Autodesk Fusion 360 part; units mm, degrees
(part 5 of 7)
sketch "Sketch93" plane through (0, 0, 13.6) normal (0, 0, -1) x (1, 0, 0)
  circle A0 centre (117.65, -41.45) radius 3.85
  circle A1 centre (102.6547, -56.4453) radius 2.35
  circle A2 centre (110.15, -33.95) radius 3.85
  circle A3 centre (117.6453, -56.4453) radius 2.35
  circle A4 centre (110.15, -48.95) radius 3.85
  circle A5 centre (102.65, -41.45) radius 3.85
  circle A6 centre (110.2363, -20.8316) radius 2.5
  circle A7 centre (110.15, -62.1) radius 2.5
  line L0 (119.9, -7.9) -> (124.4, -7.9)
  line L1 (124.4, -7.9) -> (124.4, -12.9)
  line L2 (124.4, -12.9) -> (119.9, -12.9)
  line L3 (119.9, -12.9) -> (119.9, -7.9)
  line L4 (118.9, -24.9) -> (119.9, -24.9)
  line L5 (119.9, -24.9) -> (119.9, -19.9)
  line L6 (119.9, -19.9) -> (124.4, -19.9)
  line L7 (124.4, -19.9) -> (124.4, -24.9)
  line L8 (124.4, -24.9) -> (124.4, -25.9)
  line L9 (124.4, -25.9) -> (118.9, -25.9)
  line L10 (118.9, -25.9) -> (118.9, -24.9)
  line L11 (95.9, -0.9) -> (95.9, -24.9)
  line L12 (95.9, -24.9) -> (101.9, -24.9)
  line L13 (101.9, -24.9) -> (101.9, -25.9)
  line L14 (101.9, -25.9) -> (95.9, -25.9)
  line L15 (95.9, -25.9) -> (95.9, -77.2)
  line L16 (95.9, -77.2) -> (75.9, -77.2)
  line L17 (75.9, -77.2) -> (75.9, -85.1)
  line L18 (75.9, -85.1) -> (106.4, -85.1)
  arc A8 (106.4, -85.1) -> (126.4, -65.1) centre (106.4, -65.1) ccw
  line L19 (126.4, -65.1) -> (126.4, 4.1)
  line L20 (126.4, 4.1) -> (124.4, 4.1)
  line L21 (124.4, 4.1) -> (124.4, -0.9)
  line L22 (124.4, -0.9) -> (119.9, -0.9)
  line L23 (119.9, -0.9) -> (119.9, 4.1)
  line L24 (119.9, 4.1) -> (118.9, 4.1)
  line L25 (118.9, 4.1) -> (118.9, 1.6)
  line L26 (118.9, 1.6) -> (118.9, -0.9)
  line L27 (118.9, -0.9) -> (116.4, -0.9)
  line L28 (116.4, -0.9) -> (113.9, -0.9)
  line L29 (113.9, -0.9) -> (113.9, 1.2)
  line L30 (113.9, 1.2) -> (112.9, 1.2)
  line L31 (112.9, 1.2) -> (112.9, -0.9)
  line L32 (112.9, -0.9) -> (107.9, -0.9)
  line L33 (107.9, -0.9) -> (107.9, 1.2)
  line L34 (107.9, 1.2) -> (100.8678, 1.2)
  line L35 (100.8678, 1.2) -> (100.8704, -0.9)
  line L36 (100.8704, -0.9) -> (98.4, -0.9)
  line L37 (98.4, -0.9) -> (95.9, -0.9)
  line L38 (126.4, -65.1) -> (126.4, 4.1)
  arc A9 (106.4, -85.1) -> (126.4, -65.1) centre (106.4, -65.1) ccw
  line L39 (75.9, -85.1) -> (106.4, -85.1)
  line L40 (-2, -85.1) -> (75.9, -85.1)
  line L41 (-2, -85.1) -> (-12.5, -85.1)
  arc A10 (-32.5, -65.1) -> (-12.5, -85.1) centre (-12.5, -65.1) ccw
  arc A11 (-31.5, -65.1) -> (-12.5, -84.1) centre (-12.5, -65.1) ccw
  line L42 (-12.5, -84.1) -> (-6.5, -84.1)
  line L43 (-31.5, -59.1) -> (-31.5, -65.1)
  line L44 (-32.5, -65.1) -> (-32.5, -25.2)
  line L45 (-32.5, 4.1) -> (-32.5, -25.2)
  line L46 (-31.5, 4.1) -> (-31.5, -25.9)
  line L47 (-32.5, 25.3) -> (-32.5, 4.1)
  arc A12 (-22.5, 35.3) -> (-32.5, 25.3) centre (-22.5, 25.3) ccw
  line L48 (116.4, 35.3) -> (-22.5, 35.3)
  arc A13 (126.4, 25.3) -> (116.4, 35.3) centre (116.4, 25.3) ccw
  line L49 (126.4, 4.1) -> (126.4, 25.3)
  line L50 (46.95, 35.3) -> (46.95, 14.5814) construction
  arc A14 (106.4, -84.1) -> (125.4, -65.1) centre (106.4, -65.1) ccw
  line L51 (-31.5, -59.1) -> (-31.5, -25.9)
  line L52 (-32.5, 25.3) -> (-31.5, 25.3) construction
  line L53 (-31.5, 25.3) -> (-31.5, 4.1)
  line L54 (116.4, 35.3) -> (116.4, 34.3) construction
  line L55 (116.4, 34.3) -> (-22.5, 34.3)
  arc A15 (-22.5, 34.3) -> (-31.5, 25.3) centre (-22.5, 25.3) ccw
  arc A16 (125.4, 25.3) -> (116.4, 34.3) centre (116.4, 25.3) ccw
  line L56 (125.4, 4.1) -> (125.4, -25.9)
  line L57 (125.4, 25.3) -> (125.4, 4.1)
  line L58 (125.4, -59.1) -> (125.4, -25.9)
  line L59 (125.4, -65.1) -> (125.4, -59.1)
  line L60 (106.4, -84.1) -> (-6.5, -84.1)
  line L61 (126.4, -65.1) -> (125.4, -65.1)
  line L62 (106.4, -85.1) -> (106.4, -84.1)
  line L63 (-12.5, -85.1) -> (-12.5, -84.1)
  line L64 (-32.5, -65.1) -> (-31.5, -65.1)
  line L65 (116.4, 35.3) -> (116.4, 34.3)
  line L66 (-22.5, 35.3) -> (-22.5, 34.3)
  dimension "d636" = 1
  dimension "d637" = 1
  constraint midpoint L48 L50.start
  constraint perpendicular L48 L50
  constraint symmetric A11.start L50 A14.end
  constraint symmetric A11.end L50 A14.start
  constraint symmetric A11 L50 A14
  constraint coincident L43.start L51.start
  constraint coincident L46.end L51.end
  constraint coincident L47.start A12.end
  constraint perpendicular L47 L52
  constraint concentric A12 A15
  constraint coincident L46.start L53.end
  constraint coincident L48.start A13.end
  constraint perpendicular L48 L54
  constraint tangent L55 A15
  constraint symmetric L46.start L50 L56.start
  constraint symmetric L46.end L50 L56.end
  constraint symmetric L50 L43.start L58.start
  constraint symmetric L50 L46.end L56.end
  constraint symmetric L50 L52.end A16.start
  constraint symmetric L50 L46.start L56.start
  constraint symmetric L50 L55.end L54.end
  constraint symmetric L50 A15 A16
  constraint coincident L42.end L60.end
  constraint coincident A8.end L19.start
  constraint coincident L18.end A8.start
  constraint coincident L41.end A10.end
  constraint coincident A11.end L42.start
  constraint coincident A10.start L44.start
  constraint coincident A11.start L43.end
  constraint coincident A12.start L48.end
  measures "d636" distance of L47.start L52.end
  measures "d637" distance of L48.start L54.end
extrude "Extrude79" add sketch "Sketch93" along normal blind 22 contours L19 L20 L38 L56 L58 L59 L61 | L43 L44 L45 L46 L47 A12 L51 L53 A15 L64 L66 | L20 A13 L49 A16 L57 L65 bodies 3
extrude "Extrude80" add 1 faces at (33.342, 24.9132, -5.7) along direction (0, 0, -1) blind 8 on bodies 2 bodies 2
extrude "Extrude82" add 7 faces at (126.0667, 11.9, -8.4) (114.6093, -1.7242, -8.4) (118.1907, -25.4242, -8.4) (18.7093, 81.2742, -8.4) (-20.7093, -1.7242, -8.4) (-20.7093, -25.1758, -8.4) (-31.8333, 28.7333, -8.4) along direction (0, 0, -1) blind 8 on bodies 3 bodies 3
sketch "Sketch95" plane through (-32.5, 0, 0) normal (-1, 0, 0) x (0, -1, 0)
  line L0 (25.3, -16.4) -> (25.3, 14.6)
  line L1 (25.3, 14.6) -> (4.1, 14.6)
  line L2 (4.1, 14.6) -> (4.1, 13.6)
  line L3 (4.1, 13.6) -> (-25.2, 13.6)
  line L4 (-25.2, 13.6) -> (-25.2, -16.4)
  line L5 (-25.2, -16.4) -> (25.3, -16.4)
  line L6 (-11.4882, 13.6) -> (30.9382, 13.6) construction
  line L7 (-11.4882, 13.6) -> (-13.9882, 13.6)
  line L8 (-11.4882, 13.6) -> (-8.9882, 13.6)
  line L9 (18.5118, -16.4) -> (21.0118, -16.4)
  line L10 (18.5118, -16.4) -> (16.0118, -16.4)
  line L11 (-13.9882, 13.6) -> (16.0118, -16.4)
  line L12 (-8.9882, 13.6) -> (21.0118, -16.4)
  dimension "d658" = 2.5
  dimension "d659" = 2.5
  dimension "d660" = 2.5
  dimension "d661" = 2.5
  constraint horizontal L6
  constraint coincident L3 L6.start
  constraint coincident L5 L9.start
  constraint parallel L3 L7
  constraint parallel L6 L8
  constraint parallel L5 L9
  constraint parallel L5 L10
  measures "d658" distance of L6.start L7.end
  measures "d659" distance of L6.start L8.end
  measures "d660" distance of L9.start L9.end
  measures "d661" distance of L9.start L10.end
extrude "Extrude84" add sketch "Sketch95" along normal blind 1 contours L3 L5 L7 L8 L9 L10 L11 L12 bodies 3 6 8
fillet "Fillet7" radius 5 1 edges at (-32.5, -6.0118, -1.4) on bodies 3
fillet "Fillet8" radius 8.5 1 edges at (-33.5, -6.0118, -1.4) on bodies 3
fillet "Fillet9" radius 5 1 edges at (-32.5, -1.0118, -1.4) on bodies 3
fillet "Fillet10" radius 8.5 1 edges at (-33.5, -1.0118, -1.4) on bodies 3
sketch "Sketch97" plane through (0, 0, 15.6) normal (0, 0, 1) x (-1, 0, 0)
  arc A0 (31.5, 25.3) -> (27.4749, 32.8) centre (22.5, 25.3) ccw
  line L0 (27.4749, 32.8) -> (15.9888, 32.8)
  line L1 (15.9888, 32.8) -> (17.8764, 30.7591)
  arc A1 (15.9888, 31.4975) -> (17.8764, 30.7591) centre (16.1, 29) ccw
  line L2 (15.9888, 31.4975) -> (15.9888, 32.8)
  line L3 (15.9888, 32.8) -> (-121.3749, 32.8)
  arc A2 (-121.3749, 32.8) -> (-125.4, 25.3) centre (-116.4, 25.3) ccw
  line L4 (-125.4, 25.3) -> (-125.4, -65.1)
  arc A3 (-125.4, -65.1) -> (-106.4, -84.1) centre (-106.4, -65.1) ccw
  line L5 (-106.4, -84.1) -> (12.5, -84.1)
  arc A4 (12.5, -84.1) -> (31.5, -65.1) centre (12.5, -65.1) ccw
  line L6 (31.5, -65.1) -> (31.5, -25.2)
  line L7 (31.5, -25.2) -> (31.5, 25.3)
  line L8 (0, 4.1) -> (0, -75.1)
  line L9 (0, -75.1) -> (-93.9, -75.1)
  line L10 (-93.9, -75.1) -> (-93.9, 4.1)
  line L11 (-93.9, 4.1) -> (0, 4.1)
  circle A5 centre (-102.6547, -56.4453) radius 2.35
  circle A6 centre (-117.6453, -56.4453) radius 2.35
  circle A7 centre (-110.15, -33.95) radius 3.85
  circle A8 centre (-102.65, -41.45) radius 3.85
  circle A9 centre (-117.65, -41.45) radius 3.85
  circle A10 centre (-110.15, -48.95) radius 3.85
  arc A11 (-46.45, -79.6) -> (-47.45, -79.6) centre (-46.95, -79.6) ccw
  line L12 (-46.45, -79.6) -> (-45.65, -79.6)
  arc A12 (-45.65, -80.6) -> (-45.65, -79.6) centre (-45.65, -80.1) ccw
  line L13 (-45.65, -80.6) -> (-46.45, -80.6)
  arc A13 (-47.45, -80.6) -> (-46.45, -80.6) centre (-46.95, -80.6) ccw
  line L14 (-47.45, -80.6) -> (-48.25, -80.6)
  arc A14 (-48.25, -79.6) -> (-48.25, -80.6) centre (-48.25, -80.1) ccw
  line L15 (-48.25, -79.6) -> (-47.45, -79.6)
  line L16 (-98.8996, 12.7) -> (-88.8996, 12.7)
  arc A15 (-88.9, 10.7) -> (-88.8996, 12.7) centre (-88.9, 11.7) ccw
  line L17 (-88.9, 10.7) -> (-98.9, 10.7)
  arc A16 (-98.8996, 12.7) -> (-98.9, 10.7) centre (-98.9, 11.7) ccw
  line L18 (-85.7348, 14.7) -> (-102.0652, 14.7)
  arc A17 (-102.0652, 16.7) -> (-102.0652, 14.7) centre (-102.0652, 15.7) ccw
  line L19 (-102.0652, 16.7) -> (-85.7348, 16.7)
  arc A18 (-85.7348, 14.7) -> (-85.7348, 16.7) centre (-85.7348, 15.7) ccw
  arc A19 (-102.0652, 24.7) -> (-102.0652, 22.7) centre (-102.0652, 23.7) ccw
  line L20 (-102.0652, 24.7) -> (-85.7348, 24.7)
  arc A20 (-85.7348, 22.7) -> (-85.7348, 24.7) centre (-85.7348, 23.7) ccw
  line L21 (-85.7348, 22.7) -> (-102.0652, 22.7)
  arc A21 (-98.9, 28.7) -> (-98.9004, 26.7) centre (-98.9, 27.7) ccw
  line L22 (-98.9, 28.7) -> (-88.9, 28.7)
  arc A22 (-88.8996, 26.7) -> (-88.9, 28.7) centre (-88.9, 27.7) ccw
  line L23 (-88.8996, 26.7) -> (-98.9004, 26.7)
  arc A23 (-102.9, 20.7) -> (-102.9, 18.7) centre (-102.9, 19.7) ccw
  line L24 (-102.9, 20.7) -> (-84.9, 20.7)
  arc A24 (-84.9, 18.7) -> (-84.9, 20.7) centre (-84.9, 19.7) ccw
  line L25 (-84.9, 18.7) -> (-102.9, 18.7)
  line L26 (8.1652, 14.7) -> (-8.1652, 14.7)
  arc A25 (-8.1652, 16.7) -> (-8.1652, 14.7) centre (-8.1652, 15.7) ccw
  line L27 (-8.1652, 16.7) -> (8.1652, 16.7)
  arc A26 (8.1652, 14.7) -> (8.1652, 16.7) centre (8.1652, 15.7) ccw
  arc A27 (9, 18.7) -> (9, 20.7) centre (9, 19.7) ccw
  line L28 (9, 18.7) -> (-9, 18.7)
  arc A28 (-9, 20.7) -> (-9, 18.7) centre (-9, 19.7) ccw
  line L29 (-9, 20.7) -> (9, 20.7)
  line L30 (-8.1652, 24.7) -> (8.1652, 24.7)
  arc A29 (8.1652, 22.7) -> (8.1652, 24.7) centre (8.1652, 23.7) ccw
  line L31 (8.1652, 22.7) -> (-8.1652, 22.7)
  arc A30 (-8.1652, 24.7) -> (-8.1652, 22.7) centre (-8.1652, 23.7) ccw
  arc A31 (5.0004, 26.7) -> (5, 28.7) centre (5, 27.7) ccw
  line L32 (5.0004, 26.7) -> (-4.9996, 26.7)
  arc A32 (-5, 28.7) -> (-4.9996, 26.7) centre (-5, 27.7) ccw
  line L33 (-5, 28.7) -> (5, 28.7)
  arc A33 (5, 10.7) -> (5.0004, 12.7) centre (5, 11.7) ccw
  line L34 (5, 10.7) -> (-5, 10.7)
  arc A34 (-5.0004, 12.7) -> (-5, 10.7) centre (-5, 11.7) ccw
  line L35 (-5.0004, 12.7) -> (5.0004, 12.7)
  line L36 (-34.2, 32.4) -> (-34.2, 30.4)
  line L37 (-34.2, 30.4) -> (-27.2, 30.4)
  line L38 (-27.2, 30.4) -> (-27.2, 10)
  arc A35 (-29.2, 8) -> (-27.2, 10) centre (-29.2, 10) ccw
  line L39 (-29.2, 8) -> (-64.7, 8)
  arc A36 (-66.7, 10) -> (-64.7, 8) centre (-64.7, 10) ccw
  line L40 (-66.7, 10) -> (-66.7, 30.4)
  line L41 (-66.7, 30.4) -> (-59.7, 30.4)
  line L42 (-59.7, 30.4) -> (-59.7, 32.4)
  line L43 (-59.7, 32.4) -> (-34.2, 32.4)
  line L44 (13, -32.2) -> (19.5, -32.2)
  line L45 (19.5, -32.2) -> (19.5, -38.2)
  line L46 (19.5, -38.2) -> (25.5, -38.2)
  line L47 (25.5, -38.2) -> (25.5, -44.7)
  line L48 (25.5, -44.7) -> (19.5, -44.7)
  line L49 (19.5, -44.7) -> (19.5, -50.7)
  line L50 (19.5, -50.7) -> (13, -50.7)
  line L51 (13, -50.7) -> (13, -44.7)
  line L52 (13, -44.7) -> (7, -44.7)
  line L53 (7, -44.7) -> (7, -38.2)
  line L54 (7, -38.2) -> (13, -38.2)
  line L55 (13, -38.2) -> (13, -32.2)
  circle A37 centre (10.8119, -62.3239) radius 1.5
  circle A38 centre (16.25, -62.1) radius 0.4
  line L56 (16.25, -62.1) -> (16.25, -66.288) construction
  line L57 (10.8119, -62.3239) -> (16.25, -62.3239) construction
  line L58 (16.25, -62.3239) -> (21.688, -62.3239) construction
  line L59 (21.688, -62.3239) -> (21.688, -60.8239) construction
  line L60 (20.188, -62.3239) -> (20.188, -59.3239)
  line L61 (23.188, -62.3239) -> (23.188, -59.3239)
  arc A39 (20.188, -62.3239) -> (23.188, -62.3239) centre (21.688, -62.3239) ccw
  arc A40 (23.188, -59.3239) -> (20.188, -59.3239) centre (21.688, -59.3239) ccw
  dimension "d674" = 5.438
  dimension "d675" = 3
  dimension "d676" = 3
  constraint coincident A38.centre L56.start
  constraint vertical L56
  constraint coincident A37.centre L57.start
  constraint coincident L56 L57.end
  constraint perpendicular L56 L57
  constraint perpendicular L56 L58
  constraint coincident L58.end L59.start
  constraint perpendicular L58 L59
  constraint tangent A39 A40
  constraint coincident L58 L60.start
  constraint tangent L60 A40
  constraint tangent L61 A40
  constraint parallel L60 L61
  measures "d674" distance of L57.end L58.end
  measures "d675" diameter of A39
  measures "d676" distance of L58.end A40.centre
extrude "Extrude85" cut sketch "Sketch97" against normal blind 1 contours L60 L61 A39 A40 bodies 3
sketch "Sketch98" plane through (126.4, 0, 0) normal (1, 0, 0) x (0, 1, 0)
  line L0 (65.1, 13.6) -> (65.1, 14.6)
  line L1 (65.1, 14.6) -> (-25.3, 14.6)
  line L2 (-25.3, 14.6) -> (-25.3, -16.4)
  line L3 (-25.3, -16.4) -> (65.1, -16.4)
  line L4 (65.1, -16.4) -> (65.1, 13.6)
  line L5 (-21.0118, -16.4) -> (-16.0118, -16.4)
  line L6 (13.9, 13.6) -> (8.9882, 13.6)
  line L7 (8.9882, 13.6) -> (-21.0118, -16.4)
  line L8 (13.9, 13.6) -> (-16.0118, -16.4)
  point P0 (-21.0118, -16.4)
  point P1 (-16.0118, -16.4)
  point P2 (13.9, 13.6)
  point P3 (8.9882, 13.6)
  constraint coincident P0 L5.start
  constraint coincident P1 L5.end
  constraint coincident P2 L6.start
  constraint coincident P3 L6.end
extrude "Extrude86" add sketch "Sketch98" along normal blind 1 contours L3 L5 L6 L7 L8 bodies 3 6 8
fillet "Fillet13" radius 5 1 edges at (126.4, -6.0118, -1.4) on bodies 3
fillet "Fillet14" radius 8.5 1 edges at (127.4, -6.0118, -1.4) on bodies 3
fillet "Fillet15" radius 5 1 edges at (126.4, -1.0559, -1.4) on bodies 3
fillet "Fillet16" radius 8.5 1 edges at (127.4, -1.0559, -1.4) on bodies 3
sketch "Sketch102" plane through (0, 0, 10) normal (0, 0, -1) x (1, 0, 0)
  line L0 (-31.5, 25.3) -> (-31.5, 4.1)
  line L1 (-31.5, 4.1) -> (-25, 4.1)
  line L2 (-25, 4.1) -> (-25, 1.6)
  arc A0 (-23, 4.0495) -> (-25, 1.6) centre (-22.5, 1.6) ccw
  line L3 (-23, 4.0495) -> (-23, 22.8505)
  arc A1 (-22, 22.8505) -> (-23, 22.8505) centre (-22.5, 25.3) ccw
  line L4 (-22, 22.8505) -> (-22, 4.0495)
  arc A2 (-20, 1.6) -> (-22, 4.0495) centre (-22.5, 1.6) ccw
  line L5 (-20, 1.6) -> (-20, 2)
  line L6 (-20, 2) -> (-7, 2)
  line L7 (-7, 2) -> (-7, 4.1)
  line L8 (-7, 4.1) -> (-4.5, 4.1)
  line L9 (-4.5, 4.1) -> (-2, 4.1)
  line L10 (-2, 4.1) -> (0, 4.1)
  line L11 (0, 4.1) -> (0, 5.7)
  arc A3 (13.4164, 23.7) -> (0, 5.7) centre (0, 19.7) ccw
  line L12 (13.4164, 23.7) -> (27.2, 23.7)
  line L13 (27.2, 23.7) -> (27.2, 33.9)
  line L14 (27.2, 33.9) -> (66.7, 33.9)
  line L15 (66.7, 33.9) -> (66.7, 23.7)
  line L16 (66.7, 23.7) -> (80.4836, 23.7)
  arc A4 (93.9, 5.7) -> (80.4836, 23.7) centre (93.9, 19.7) ccw
  line L17 (93.9, 5.7) -> (93.9, 4.1)
  line L18 (93.9, 4.1) -> (95.9, 4.1)
  line L19 (95.9, 4.1) -> (98.4, 4.1)
  line L20 (98.4, 4.1) -> (100.9, 4.1)
  line L21 (100.9, 4.1) -> (100.9, 2)
  line L22 (100.9, 2) -> (113.9322, 2)
  arc A5 (115.9, 4.0495) -> (113.9322, 2) centre (116.4, 1.6) ccw
  line L23 (115.9, 4.0495) -> (115.9, 22.8505)
  arc A6 (116.9, 22.8505) -> (115.9, 22.8505) centre (116.4, 25.3) ccw
  line L24 (116.9, 22.8505) -> (116.9, 4.0495)
  arc A7 (118.9, 1.6) -> (116.9, 4.0495) centre (116.4, 1.6) ccw
  line L25 (118.9, 1.6) -> (118.9, 4.1)
  line L26 (118.9, 4.1) -> (125.4, 4.1)
  line L27 (125.4, 4.1) -> (125.4, 25.3)
  arc A8 (125.4, 25.3) -> (116.4, 34.3) centre (116.4, 25.3) ccw
  line L28 (116.4, 34.3) -> (116.4, 35.3)
  line L29 (116.4, 35.3) -> (-22.5, 35.3)
  line L30 (-22.5, 35.3) -> (-22.5, 34.3)
  arc A9 (-22.5, 34.3) -> (-31.5, 25.3) centre (-22.5, 25.3) ccw
  line L31 (116.4, 35.3) -> (96.4, 35.3)
  line L32 (96.4, 35.3) -> (96.4, 34.3)
  line L33 (96.4, 34.3) -> (116.4, 34.3)
  line L34 (116.4, 34.3) -> (116.4, 35.3)
  line L35 (46.95, 35.3) -> (46.95, 48.5522) construction
  line L36 (46.95, 35.3) -> (46.95, 48.5522) construction
  line L37 (-22.5, 35.3) -> (-2.5, 35.3)
  line L38 (-2.5, 35.3) -> (-2.5, 34.3)
  line L39 (-2.5, 34.3) -> (-22.5, 34.3)
  line L40 (-22.5, 34.3) -> (-22.5, 35.3)
  dimension "d693" = 20
  dimension "d694" = 1
  constraint coincident L28.end L29.start
  constraint perpendicular L28 L31
  constraint perpendicular L31 L32
  constraint coincident A8.end L28.start
  constraint midpoint L29 L35.start
  constraint perpendicular L29 L35
  constraint symmetric L28.end L35 L29.end
  constraint symmetric L31.end L35 L37.end
  constraint symmetric L32.end L35 L38.end
  constraint symmetric A8.end L35 L30.end
  constraint symmetric L36.start L35 L35.start
  constraint symmetric L36.end L35 L35.end
  measures "d693" distance of L28.end L31.end
  measures "d694" distance of L31.end L32.end
extrude "Extrude87" add sketch "Sketch102" along normal blind 26.4 contours L29 L30 L37 L38 L39 L40 | L28 L29 L31 L32 L33 L34 bodies 3 6 8
sketch "ExportDXF" plane through (0, 0, -16.4) normal (0, 0, -1) x (1, 0, 0)
  circle A0 centre (116.4, 1.6) radius 0.4
  circle A1 centre (116.4, 1.6) radius 2.5
  spline S0 degree 3 poles (121.3749, 32.8) (121.4016, 32.8) (121.4257, 32.8021) (121.4681, 32.811) (121.489, 32.8182) (121.521, 32.8394) (121.5326, 32.8506) (121.5513, 32.8783) (121.5579, 32.8938) (121.5687, 32.9351) (121.5705, 32.9623) (121.568, 33.0372) (121.5571, 33.0944) (121.5047, 33.2719) (121.442, 33.4168) (121.2247, 33.772) (121.0595, 33.976) (120.605, 34.3502) (120.3486, 34.4924) (120.0657, 34.6039) knots 1.719139 1.719139 1.719139 1.719139 1.741292 1.741292 1.762806 1.762806 1.778603 1.778603 1.794207 1.794207 1.817491 1.817491 1.860621 1.860621 1.939646 1.939646 2.038469 2.038469 2.13754 2.13754 2.13754 2.13754
  arc A2 (126.4, 25.3) -> (120.0657, 34.6039) centre (116.4, 25.3) ccw
  line L0 (126.4, 25.3) -> (125.4, 25.3)
  arc A3 (125.4, 25.3) -> (121.3749, 32.8) centre (116.4, 25.3) ccw
  circle A4 centre (98.4, 1.6) radius 0.4
  circle A5 centre (110.2363, -20.8316) radius 2.5
  circle A6 centre (110.2363, -20.8316) radius 2.5
  line L1 (115.9, 22.8505) -> (115.9, 4.0495)
  line L2 (115.9, 4.0495) -> (115.9, 22.8505)
  circle A7 centre (102.6547, -56.4453) radius 2.35
  circle A8 centre (102.6547, -56.4453) radius 2.35
  line L3 (-25, 1.6) -> (-25, -0.9)
  line L4 (-25, -0.9) -> (-25, 1.6)
  circle A9 centre (117.6453, -56.4453) radius 2.35
  circle A10 centre (117.6453, -56.4453) radius 2.35
  circle A11 centre (98.4, 1.6) radius 0.4
  circle A12 centre (98.4, 1.6) radius 0.4
  circle A13 centre (116.4, 25.3) radius 0.4
  circle A14 centre (116.4, 25.3) radius 2.5
  arc A15 (106.4, -85.1) -> (126.4, -65.1) centre (106.4, -65.1) ccw
  arc A16 (106.4, -85.1) -> (126.4, -65.1) centre (106.4, -65.1) ccw
  line L5 (96.4, 34.3) -> (116.4, 34.3)
  line L6 (116.4, 34.3) -> (96.4, 34.3)
  line L7 (-22.4996, -0.9) -> (-25, -0.9)
  line L8 (-25, -0.9) -> (-22.4996, -0.9)
  line L9 (-25, 4.1) -> (-25, 1.6)
  line L10 (-25, 1.6) -> (-25, 4.1)
  circle A17 centre (116.4, 1.6) radius 2.5
  arc A18 (113.9322, 2) -> (113.9322, 1.2) centre (116.4, 1.6) ccw
  arc A19 (113.9322, 1.2) -> (116.4, -0.9) centre (116.4, 1.6) ccw
  arc A20 (116.4, -0.9) -> (118.9, 1.6) centre (116.4, 1.6) ccw
  arc A21 (118.9, 1.6) -> (116.9, 4.0495) centre (116.4, 1.6) ccw
  arc A22 (116.9, 4.0495) -> (115.9, 4.0495) centre (116.4, 1.6) ccw
  arc A23 (115.9, 4.0495) -> (113.9322, 2) centre (116.4, 1.6) ccw
  line L11 (-26, 4.1) -> (-26, -0.9)
  line L12 (-26, -0.9) -> (-26, 4.1)
  circle A24 centre (116.4, 1.6) radius 0.4
  arc A25 (116.4, 2) -> (116.3992, 1.2) centre (116.4, 1.6) ccw
  arc A26 (116.3992, 1.2) -> (116.4, 2) centre (116.4, 1.6) ccw
  circle A27 centre (110.2363, -20.8316) radius 0.4
  circle A28 centre (110.2363, -20.8316) radius 2.5
  line L13 (116.9, 4.0495) -> (116.9, 22.8505)
  line L14 (116.9, 22.8505) -> (116.9, 4.0495)
  line L15 (125.4, 4.1) -> (118.9, 4.1)
  line L16 (118.9, 4.1) -> (119.9, 4.1)
  line L17 (119.9, 4.1) -> (124.4, 4.1)
  line L18 (124.4, 4.1) -> (125.4, 4.1)
  line L19 (-19, -6.9) -> (-14, -6.9)
  line L20 (-14, -6.9) -> (-14, -1.9)
  line L21 (-14, -1.9) -> (-19, -1.9)
  line L22 (-19, -1.9) -> (-19, -6.9)
  arc A29 (113.9322, 2) -> (113.9322, 1.2) centre (116.4, 1.6) ccw
  line L23 (113.9322, 2) -> (100.9, 2)
  line L24 (100.9, 2) -> (100.9, 1.6)
  arc A30 (100.8678, 1.2) -> (100.9, 1.6) centre (98.4, 1.6) ccw
  line L25 (100.8678, 1.2) -> (113.9322, 1.2)
  arc A31 (125.4, 25.3) -> (116.4, 34.3) centre (116.4, 25.3) ccw
  arc A32 (125.4, 25.3) -> (116.4, 34.3) centre (116.4, 25.3) ccw
  line L26 (-30.5, 4.1) -> (-30.5, -0.9)
  line L27 (-30.5, -0.9) -> (-26, -0.9)
  line L28 (-26, -0.9) -> (-26, 4.1)
  line L29 (-26, 4.1) -> (-30.5, 4.1)
  line L30 (113.9322, 2) -> (100.9, 2)
  line L31 (100.9, 2) -> (113.9322, 2)
  line L32 (-25, 1.6) -> (-25, -0.9)
  line L33 (-25, -0.9) -> (-22.4996, -0.9)
  arc A33 (-25, 1.6) -> (-22.4996, -0.9) centre (-22.5, 1.6) ccw
  line L34 (-26, -6.9) -> (-26, -1.9)
  line L35 (-26, -1.9) -> (-30.5, -1.9)
  line L36 (-30.5, -1.9) -> (-30.5, -6.9)
  line L37 (-30.5, -6.9) -> (-26, -6.9)
  line L38 (117.9635, 35.177) -> (116.4, 35.177)
  line L39 (116.4, 35.177) -> (116.4, 35.3)
  arc A34 (117.9635, 35.177) -> (116.4, 35.3) centre (116.4, 25.3) ccw
  arc A35 (100.8678, 1.2) -> (100.9, 1.6) centre (98.4, 1.6) ccw
  arc A36 (98.4, -0.9) -> (100.9, 1.6) centre (98.4, 1.6) ccw
  arc A37 (98.4, -0.9) -> (100.8678, 1.2) centre (98.4, 1.6) ccw
  line L40 (-20, -6.9) -> (-20, -1.9)
  line L41 (-20, -1.9) -> (-25, -1.9)
  line L42 (-25, -1.9) -> (-25, -6.9)
  line L43 (-25, -6.9) -> (-20, -6.9)
  line L44 (116.4, 35.3) -> (116.4, 35.177)
  line L45 (116.4, 35.3) -> (116.4, 35.177)
  line L46 (100.9, 2) -> (100.9, 4.1)
  line L47 (100.9, 4.1) -> (100.9, 1.6)
  line L48 (100.9, 1.6) -> (100.9, 2)
  line L49 (125.4, 25.3) -> (125.4, 4.1)
  line L50 (125.4, 4.1) -> (125.4, 25.3)
  arc A38 (112.3364, -53.5022) -> (114.4671, -46.3299) centre (110.15, -48.95) ccw
  arc A39 (112.3364, -53.5022) -> (114.4671, -46.3299) centre (110.15, -48.95) ccw
  circle A40 centre (-16.1626, -20.3028) radius 0.4
  line L51 (-25, -6.9) -> (-25, -1.9)
  line L52 (-25, -1.9) -> (-25, -6.9)
  circle A41 centre (-16.1626, -20.3028) radius 0.4
  circle A42 centre (-16.1626, -20.3028) radius 2.5
  spline S1 degree 3 poles (126.7177, -15.6596) (127.0784, -14.2999) (127.2562, -12.8809) (127.2612, -10.0454) (127.0837, -8.6064) (126.7183, -7.2283) knots 0 0 0 0 0.422012 0.422012 0.849727 0.849727 0.849727 0.849727
  line L53 (126.7183, -7.2283) -> (126.7227, 22.7553)
  spline S2 degree 3 poles (126.7227, 22.7553) (127.0885, 21.3861) (127.2684, 19.9562) (127.2724, 17.1016) (127.0924, 15.654) (126.7221, 14.2685) knots 0 0 0 0 0.425176 0.425176 0.855407 0.855407 0.855407 0.855407
  line L54 (126.7221, 14.2685) -> (126.7177, -15.6596)
  circle A43 centre (102.6547, -56.4453) radius 5
  circle A44 centre (102.6547, -56.4453) radius 2.35
  line L55 (-26, -0.9) -> (-30.5, -0.9)
  line L56 (-30.5, -0.9) -> (-26, -0.9)
  circle A45 centre (110.15, -48.95) radius 3.85
  circle A46 centre (110.15, -48.95) radius 3.85
  arc A47 (126.4, 25.3) -> (120.0657, 34.6039) centre (116.4, 25.3) ccw
  spline S3 degree 3 poles (120.0657, 34.6039) (119.5111, 34.8224) (118.9454, 34.9877) (118.2417, 35.13) (118.1027, 35.155) (117.9635, 35.177) knots -0.429091 -0.429091 -0.429091 -0.429091 -0.227456 -0.227456 -0.177677 -0.177677 -0.177677 -0.177677
  arc A48 (117.9635, 35.177) -> (116.4, 35.3) centre (116.4, 25.3) ccw
  arc A49 (126.4, 25.3) -> (116.4, 35.3) centre (116.4, 25.3) ccw
  line L57 (95.9, -0.9) -> (98.4, -0.9)
  line L58 (98.4, -0.9) -> (95.9, -0.9)
  line L59 (-25, -1.9) -> (-20, -1.9)
  line L60 (-20, -1.9) -> (-25, -1.9)
  circle A50 centre (117.6453, -56.4453) radius 5
  circle A51 centre (117.6453, -56.4453) radius 2.35
  line L61 (-30.5, -0.9) -> (-30.5, 4.1)
  line L62 (-30.5, 4.1) -> (-30.5, -0.9)
  line L63 (100.8678, 1.2) -> (107.9, 1.2)
  line L64 (107.9, 1.2) -> (112.9, 1.2)
  line L65 (112.9, 1.2) -> (113.9, 1.2)
  line L66 (113.9, 1.2) -> (113.9322, 1.2)
  line L67 (113.9322, 1.2) -> (100.8678, 1.2)
  line L68 (126.7221, 14.2685) -> (126.7177, -15.6596)
  ellipse E0 centre (131.4, 11.7754) end of major axis (131.4, 18.8361) minor radius 5 (126.7221, 14.2685) -> (126.4, 11.7754) ccw
  line L69 (126.4, 11.7754) -> (126.4, -18.1364)
  ellipse E1 centre (131.4, -18.1364) end of major axis (131.4, -11.0757) minor radius 5 (126.7177, -15.6596) -> (126.4, -18.1364) ccw
  line L70 (-20, -6.9) -> (-25, -6.9)
  line L71 (-25, -6.9) -> (-20, -6.9)
  line L72 (126.7183, -7.2283) -> (126.7227, 22.7553)
  ellipse E2 centre (131.4, -4.7455) end of major axis (131.4, -11.8166) minor radius 5 (126.4, -4.7455) -> (126.7183, -7.2283) ccw
  line L73 (126.4, -4.7455) -> (126.4, 25.2545)
  ellipse E3 centre (131.4, 25.2545) end of major axis (131.4, 18.1834) minor radius 5 (126.4, 25.2545) -> (126.7227, 22.7553) ccw
  line L74 (-6.979, -7.9) -> (-2, -7.9)
  line L75 (-2, -7.9) -> (-6.979, -7.9)
  line L76 (27.2, 10) -> (27.2, 4.1)
  line L77 (27.2, 4.1) -> (66.7, 4.1)
  line L78 (66.7, 4.1) -> (66.7, 10)
  arc A52 (64.7, 8) -> (66.7, 10) centre (64.7, 10) ccw
  line L79 (64.7, 8) -> (29.2, 8)
  arc A53 (27.2, 10) -> (29.2, 8) centre (29.2, 10) ccw
  line L80 (-31.5, -59.1) -> (-31.5, -65.1)
  line L81 (-31.5, -65.1) -> (-31.5, -59.1)
  line L82 (-30.4722, -66.1) -> (-21.2419, -66.1)
  line L83 (-21.2419, -66.1) -> (-30.4722, -66.1)
  line L84 (105.6552, -46.1523) -> (107.3523, -44.4552)
  line L85 (107.3523, -44.4552) -> (105.6552, -46.1523)
  line L86 (0, -27.1) -> (-2, -27.1)
  line L87 (-2, -27.1) -> (0, -27.1)
  circle A54 centre (20.5, -81.15) radius 2.5
  arc A55 (18, -81.15) -> (23, -81.15) centre (20.5, -81.15) ccw
  arc A56 (23, -81.15) -> (18, -81.15) centre (20.5, -81.15) ccw
  line L88 (0, -71.1) -> (0, -27.1)
  line L89 (0, -27.1) -> (-2, -27.1)
  line L90 (-2, -27.1) -> (-2, -71.1)
  line L91 (-2, -71.1) -> (0, -71.1)
  circle A57 centre (102.65, -41.45) radius 3.85
  circle A58 centre (102.65, -41.45) radius 3.85
  line L92 (-5, -75) -> (-5, -57)
  line L93 (-5, -57) -> (-5, -75)
  arc A59 (-10.1676, -38.2) -> (-13, -35.3676) centre (-16.25, -41.45) ccw
  arc A60 (-10.1676, -38.2) -> (-13, -35.3676) centre (-16.25, -41.45) ccw
  arc A61 (88.8996, 12.7) -> (88.9, 10.7) centre (88.9, 11.7) ccw
  arc A62 (88.8996, 12.7) -> (88.9, 10.7) centre (88.9, 11.7) ccw
  arc A63 (107.5299, -38.2671) -> (107.9591, -38.5) centre (110.15, -33.95) ccw
  arc A64 (107.5299, -38.2671) -> (107.9591, -38.5) centre (110.15, -33.95) ccw
  line L94 (-5, -57) -> (-6, -57)
  line L95 (-6, -57) -> (-5, -57)
  line L96 (-6, -57) -> (-6, -75)
  line L97 (-6, -75) -> (-6, -57)
  arc A65 (107.185, -39.2283) -> (98.0852, -39.29) centre (102.65, -41.45) ccw
  arc A66 (107.185, -39.2283) -> (98.0852, -39.29) centre (102.65, -41.45) ccw
  line L98 (-13, -38.2) -> (-10.1676, -38.2)
  arc A67 (-10.1676, -38.2) -> (-13, -35.3676) centre (-16.25, -41.45) ccw
  line L99 (-13, -35.3676) -> (-13, -38.2)
  line L100 (23, -81.15) -> (23, -77.2)
  line L101 (23, -77.2) -> (23, -81.15)
  line L102 (-6.9716, -1.9) -> (-2, -1.9)
  line L103 (-2, -1.9) -> (-6.9716, -1.9)
  line L104 (27.2, 33.9) -> (27.2, 30.4)
  line L105 (27.2, 30.4) -> (34.2, 30.4)
  line L106 (34.2, 30.4) -> (34.2, 32.4)
  line L107 (34.2, 32.4) -> (59.7, 32.4)
  line L108 (59.7, 32.4) -> (59.7, 30.4)
  line L109 (59.7, 30.4) -> (66.7, 30.4)
  line L110 (66.7, 30.4) -> (66.7, 33.9)
  line L111 (66.7, 33.9) -> (27.2, 33.9)
  arc A68 (-9.5307, -34.5574) -> (-22.9827, -34.7173) centre (-16.25, -35.2) ccw
  arc A69 (-9.5307, -34.5574) -> (-22.9827, -34.7173) centre (-16.25, -35.2) ccw
  line L112 (-30.5, -60.1) -> (-25.5, -65.1)
  line L113 (-25.5, -65.1) -> (-30.5, -60.1)
  arc A70 (-22.9827, -34.7173) -> (-22.9827, -48.1827) centre (-22.5, -41.45) ccw
  arc A71 (-22.9827, -34.7173) -> (-22.9827, -48.1827) centre (-22.5, -41.45) ccw
  line L114 (-6.9778, -6.9) -> (-6.9716, -1.9)
  line L115 (-6.9716, -1.9) -> (-6.9778, -6.9)
  arc A72 (-13, -47.5324) -> (-10.1676, -44.7) centre (-16.25, -41.45) ccw
  arc A73 (-13, -47.5324) -> (-10.1676, -44.7) centre (-16.25, -41.45) ccw
  circle A74 centre (20.5, -81.15) radius 0.4
  circle A75 centre (20.5, -81.15) radius 0.4
  line L116 (-30.5, -65.1) -> (-30.5, -60.1)
  line L117 (-30.5, -60.1) -> (-30.5, -65.1)
  circle A76 centre (-10.8119, -62.3239) radius 1.5
  circle A77 centre (-10.8119, -62.3239) radius 1.5
  line L118 (-28.5, -52.1) -> (-28.5, -61.1)
  line L119 (-28.5, -61.1) -> (-28.5, -52.1)
  line L120 (75.9, -85.1) -> (75.9, -77.2)
  line L121 (75.9, -77.2) -> (75.9, -81.15)
  line L122 (75.9, -81.15) -> (75.9, -85.1)
  line L123 (-5, -57) -> (-6, -57)
  line L124 (-6, -57) -> (-6, -75)
  line L125 (-6, -75) -> (-5, -75)
  line L126 (-5, -75) -> (-5, -57)
  line L127 (106.9671, -44.0701) -> (107.3523, -44.4552)
  line L128 (107.3523, -44.4552) -> (106.9671, -44.0701)
  line L129 (-6, -75) -> (-5, -75)
  line L130 (-5, -75) -> (-6, -75)
  arc A78 (-23.188, -62.3239) -> (-20.188, -62.3239) centre (-21.688, -62.3239) ccw
  arc A79 (-23.188, -62.3239) -> (-20.188, -62.3239) centre (-21.688, -62.3239) ccw
  line L131 (27.2, 33.9) -> (66.7, 33.9)
  line L132 (66.7, 33.9) -> (27.2, 33.9)
  line L133 (-2, -6.9) -> (-6.9778, -6.9)
  line L134 (-6.9778, -6.9) -> (-2, -6.9)
  line L135 (107.5299, -38.2671) -> (107.1448, -38.6523)
  line L136 (107.1448, -38.6523) -> (107.5299, -38.2671)
  arc A80 (-22.9827, -48.1827) -> (-9.5307, -48.3426) centre (-16.25, -47.7) ccw
  arc A81 (-22.9827, -48.1827) -> (-9.5307, -48.3426) centre (-16.25, -47.7) ccw
  line L137 (-27.5, -62.1) -> (-24.5, -65.1)
  line L138 (-24.5, -65.1) -> (-27.5, -62.1)
  line L139 (105.4477, -36.9552) -> (107.1448, -38.6523)
  line L140 (107.1448, -38.6523) -> (105.4477, -36.9552)
  line L141 (105.8329, -36.5701) -> (105.4477, -36.9552)
  line L142 (105.4477, -36.9552) -> (105.8329, -36.5701)
  circle A82 centre (110.15, -33.95) radius 3.85
  circle A83 centre (110.15, -33.95) radius 3.85
  line L143 (-6.5, -84.1) -> (-6.5, -83.1)
  line L144 (-6.5, -83.1) -> (-6.5, -84.1)
  line L145 (-13, -44.7) -> (-13, -47.5324)
  arc A84 (-13, -47.5324) -> (-10.1676, -44.7) centre (-16.25, -41.45) ccw
  line L146 (-10.1676, -44.7) -> (-13, -44.7)
  line L147 (-25.5, -65.1) -> (-30.5, -65.1)
  line L148 (-30.5, -65.1) -> (-25.5, -65.1)
  line L149 (-27.5, -62.1) -> (-27.5, -52.1)
  line L150 (-27.5, -52.1) -> (-27.5, -62.1)
  line L151 (105.2701, -45.7671) -> (105.6552, -46.1523)
  line L152 (105.6552, -46.1523) -> (105.2701, -45.7671)
  arc A85 (85.7348, 16.7) -> (85.7348, 14.7) centre (85.7348, 15.7) ccw
  arc A86 (85.7348, 16.7) -> (85.7348, 14.7) centre (85.7348, 15.7) ccw
  arc A87 (106.9671, -44.0701) -> (107.2148, -43.61) centre (102.65, -41.45) ccw
  arc A88 (106.9671, -44.0701) -> (107.2148, -43.61) centre (102.65, -41.45) ccw
  arc A89 (98.115, -43.6717) -> (105.2701, -45.7671) centre (102.65, -41.45) ccw
  arc A90 (98.115, -43.6717) -> (105.2701, -45.7671) centre (102.65, -41.45) ccw
  line L153 (0, -71.1) -> (-2, -71.1)
  line L154 (-2, -71.1) -> (0, -71.1)
  line L155 (-6.9852, -12.9) -> (-6.979, -7.9)
  line L156 (-6.979, -7.9) -> (-6.9852, -12.9)
  arc A91 (85.7348, 24.7) -> (85.7348, 22.7) centre (85.7348, 23.7) ccw
  arc A92 (85.7348, 24.7) -> (85.7348, 22.7) centre (85.7348, 23.7) ccw
  line L157 (-30.5, -59.1) -> (-31.5, -59.1)
  line L158 (-31.5, -59.1) -> (-30.5, -59.1)
  line L159 (98.0852, -39.29) -> (98.115, -43.6717)
  line L160 (98.115, -43.6717) -> (98.0852, -39.29)
  line L161 (-28.5, -61.1) -> (-30.5, -59.1)
  line L162 (-30.5, -59.1) -> (-28.5, -61.1)
  arc A93 (88.9, 28.7) -> (88.8996, 26.7) centre (88.9, 27.7) ccw
  arc A94 (88.9, 28.7) -> (88.8996, 26.7) centre (88.9, 27.7) ccw
  line L163 (-2, -12.9) -> (-6.9852, -12.9)
  line L164 (-6.9852, -12.9) -> (-2, -12.9)
  arc A95 (107.9591, -29.4) -> (105.8329, -36.5701) centre (110.15, -33.95) ccw
  arc A96 (107.9591, -29.4) -> (105.8329, -36.5701) centre (110.15, -33.95) ccw
  line L165 (-25.5, -65.1) -> (-30.5, -60.1)
  line L166 (-30.5, -60.1) -> (-30.5, -65.1)
  line L167 (-30.5, -65.1) -> (-25.5, -65.1)
  line L168 (-6.9864, -13.9) -> (-2, -13.9)
  line L169 (-2, -13.9) -> (-6.9864, -13.9)
  circle A97 centre (20.5, -81.15) radius 0.4
  circle A98 centre (20.5, -81.15) radius 2.5
  line L170 (-19.8023, -65.1) -> (-24.5, -65.1)
  line L171 (-24.5, -65.1) -> (-19.8023, -65.1)
  arc A99 (84.9, 20.7) -> (84.9, 18.7) centre (84.9, 19.7) ccw
  arc A100 (84.9, 20.7) -> (84.9, 18.7) centre (84.9, 19.7) ccw
  line L172 (66.7, 4.5) -> (66.7, 33.9)
  line L173 (66.7, 33.9) -> (66.7, 4.5)
  line L174 (0, -71.1) -> (0, -75.1)
  line L175 (0, -75.1) -> (0, 4.1)
  line L176 (0, 4.1) -> (0, 5.7)
  line L177 (0, 5.7) -> (0, 4.1)
  line L178 (0, 4.1) -> (0, -27.1)
  line L179 (0, -27.1) -> (0, -71.1)
  line L180 (24.5, -77.2) -> (16.5, -77.2)
  line L181 (16.5, -77.2) -> (24.5, -77.2)
  circle A101 centre (98.4, 1.6) radius 1
  circle A102 centre (98.4, 1.6) radius 1
  arc A103 (62.7, 9.5) -> (65.7, 12.5) centre (62.7, 12.5) ccw
  arc A104 (62.7, 9.5) -> (65.7, 12.5) centre (62.7, 12.5) ccw
  circle A105 centre (8, -81.15) radius 1
  circle A106 centre (8, -81.15) radius 1
  circle A107 centre (-4.5, 1.6) radius 0.4
  line L182 (-2, -27.1) -> (0, -27.1)
  line L183 (0, -27.1) -> (0, 4.1)
  line L184 (0, 4.1) -> (-4.5, 4.1)
  line L185 (-4.5, 4.1) -> (-7, 4.1)
  line L186 (-7, 4.1) -> (-7, 1.6)
  arc A108 (-7, 1.6) -> (-4.5, -0.9) centre (-4.5, 1.6) ccw
  line L187 (-4.5, -0.9) -> (-2, -0.9)
  line L188 (-2, -0.9) -> (-2, -27.1)
  line L189 (28.2, 25.9) -> (28.2, 12.5)
  line L190 (28.2, 12.5) -> (28.2, 25.9)
  line L191 (27.2, 33.9) -> (27.2, 4.5)
  line L192 (27.2, 4.5) -> (27.2, 33.9)
  line L193 (95.9, -71.1) -> (93.9, -71.1)
  line L194 (93.9, -71.1) -> (93.9, -75.1)
  line L195 (93.9, -75.1) -> (0, -75.1)
  line L196 (0, -75.1) -> (0, -71.1)
  line L197 (0, -71.1) -> (-2, -71.1)
  line L198 (-2, -71.1) -> (-2, -77.2)
  line L199 (-2, -77.2) -> (5.5, -77.2)
  line L200 (5.5, -77.2) -> (5.5, -81.15)
  arc A109 (5.5, -81.15) -> (10.5, -81.15) centre (8, -81.15) ccw
  line L201 (10.5, -81.15) -> (10.5, -77.2)
  line L202 (10.5, -77.2) -> (18, -77.2)
  line L203 (18, -77.2) -> (18, -81.15)
  arc A110 (23, -81.15) -> (18, -81.15) centre (20.5, -81.15) ccw
  line L204 (23, -81.15) -> (23, -77.2)
  line L205 (23, -77.2) -> (46.4092, -77.2)
  arc A111 (47.4908, -77.2) -> (46.4092, -77.2) centre (46.95, -80.1) ccw
  line L206 (47.4908, -77.2) -> (70.9, -77.2)
  line L207 (70.9, -77.2) -> (70.9, -81.15)
  arc A112 (70.9, -81.15) -> (75.9, -81.15) centre (73.4, -81.15) ccw
  line L208 (75.9, -81.15) -> (75.9, -77.2)
  line L209 (75.9, -77.2) -> (95.9, -77.2)
  line L210 (95.9, -77.2) -> (95.9, -71.1)
  circle A113 centre (73.4, -81.15) radius 0.4
  circle A114 centre (8, -81.15) radius 0.4
  line L211 (100.9, 4.1) -> (-7, 4.1)
  line L212 (-7, 4.1) -> (100.9, 4.1)
  line L213 (126.4, -65.1) -> (125.4, -65.1)
  line L214 (125.4, -65.1) -> (125.4, 4.1)
  line L215 (125.4, 4.1) -> (124.4, 4.1)
  line L216 (124.4, 4.1) -> (124.4, -0.9)
  line L217 (124.4, -0.9) -> (119.9, -0.9)
  line L218 (119.9, -0.9) -> (119.9, 4.1)
  line L219 (119.9, 4.1) -> (118.9, 4.1)
  line L220 (118.9, 4.1) -> (118.9, 1.6)
  line L221 (118.9, 1.6) -> (118.9, -0.9)
  line L222 (118.9, -0.9) -> (116.4, -0.9)
  line L223 (116.4, -0.9) -> (113.9, -0.9)
  line L224 (113.9, -0.9) -> (113.9, 1.2)
  line L225 (113.9, 1.2) -> (112.9, 1.2)
  line L226 (112.9, 1.2) -> (112.9, -0.9)
  line L227 (112.9, -0.9) -> (107.9, -0.9)
  line L228 (107.9, -0.9) -> (107.9, 1.2)
  line L229 (107.9, 1.2) -> (100.8678, 1.2)
  line L230 (100.8678, 1.2) -> (100.8704, -0.9)
  line L231 (100.8704, -0.9) -> (98.4, -0.9)
  line L232 (98.4, -0.9) -> (95.9, -0.9)
  line L233 (95.9, -0.9) -> (95.9, -24.9)
  line L234 (95.9, -24.9) -> (101.9, -24.9)
  line L235 (101.9, -24.9) -> (101.9, -25.9)
  line L236 (101.9, -25.9) -> (95.9, -25.9)
  line L237 (95.9, -25.9) -> (95.9, -77.2)
  line L238 (95.9, -77.2) -> (75.9, -77.2)
  line L239 (75.9, -77.2) -> (75.9, -85.1)
  line L240 (75.9, -85.1) -> (106.4, -85.1)
  arc A115 (106.4, -85.1) -> (126.4, -65.1) centre (106.4, -65.1) ccw
  line L241 (118.9, -24.9) -> (119.9, -24.9)
  line L242 (119.9, -24.9) -> (119.9, -19.9)
  line L243 (119.9, -19.9) -> (124.4, -19.9)
  line L244 (124.4, -19.9) -> (124.4, -24.9)
  line L245 (124.4, -24.9) -> (124.4, -25.9)
  line L246 (124.4, -25.9) -> (118.9, -25.9)
  line L247 (118.9, -25.9) -> (118.9, -24.9)
  line L248 (119.9, -7.9) -> (124.4, -7.9)
  line L249 (124.4, -7.9) -> (124.4, -12.9)
  line L250 (124.4, -12.9) -> (119.9, -12.9)
  line L251 (119.9, -12.9) -> (119.9, -7.9)
  circle A116 centre (110.15, -62.1) radius 2.5
  circle A117 centre (110.2363, -20.8316) radius 2.5
  circle A118 centre (102.65, -41.45) radius 3.85
  circle A119 centre (110.15, -48.95) radius 3.85
  circle A120 centre (117.6453, -56.4453) radius 2.35
  circle A121 centre (110.15, -33.95) radius 3.85
  circle A122 centre (102.6547, -56.4453) radius 2.35
  circle A123 centre (117.65, -41.45) radius 3.85
  arc A124 (28.2, 12.5) -> (31.2, 9.5) centre (31.2, 12.5) ccw
  line L252 (28.2, 12.5) -> (28.2, 25.9)
  arc A125 (31.2, 28.9) -> (28.2, 25.9) centre (31.2, 25.9) ccw
  line L253 (31.2, 28.9) -> (62.7, 28.9)
  arc A126 (65.7, 25.9) -> (62.7, 28.9) centre (62.7, 25.9) ccw
  line L254 (65.7, 25.9) -> (65.7, 12.5)
  arc A127 (62.7, 9.5) -> (65.7, 12.5) centre (62.7, 12.5) ccw
  line L255 (62.7, 9.5) -> (31.2, 9.5)
  circle A128 centre (73.4, -81.15) radius 1
  circle A129 centre (73.4, -81.15) radius 1
  line L256 (-27.8571, -74.4894) -> (-21.6425, -74.1949)
  line L257 (-21.6425, -74.1949) -> (-22.0173, -80.3781)
  arc A130 (-27.8571, -74.4894) -> (-22.0173, -80.3781) centre (-12.5, -65.1) ccw
  line L258 (-25.5, -65.1) -> (-30.5, -65.1)
  line L259 (-30.5, -65.1) -> (-30.5, -60.1)
  line L260 (-30.5, -60.1) -> (-25.5, -65.1)
  line L261 (-21.0008, -80.1355) -> (-20.6378, -74.1472)
  line L262 (-20.6378, -74.1472) -> (-14.7326, -73.8674)
  line L263 (-14.7326, -73.8674) -> (-21.0008, -80.1355)
  line L264 (-20.617, -81.166) -> (-13.5, -74.049)
  line L265 (-13.5, -74.049) -> (-13.5, -83.0722)
  arc A131 (-20.617, -81.166) -> (-13.5, -83.0722) centre (-12.5, -65.1) ccw
  line L266 (-20.5769, -73.1432) -> (-20.2671, -68.0326)
  arc A132 (-20.2671, -68.0326) -> (-15.3557, -72.8958) centre (-12.5, -65.1) ccw
  line L267 (-15.3557, -72.8958) -> (-20.5769, -73.1432)
  line L268 (-12.5, -78.1) -> (-7.5, -83.1)
  line L269 (-7.5, -83.1) -> (-12.5, -83.1)
  line L270 (-12.5, -83.1) -> (-12.5, -78.1)
  line L271 (-21.5816, -73.1909) -> (-27.6189, -73.477)
  line L272 (-27.6189, -73.477) -> (-21.2106, -67.0687)
  line L273 (-21.2106, -67.0687) -> (-21.5816, -73.1909)
  arc A133 (-30.4722, -66.1) -> (-28.496, -73.3541) centre (-12.5, -65.1) ccw
  line L274 (-30.4722, -66.1) -> (-21.2419, -66.1)
  line L275 (-21.2419, -66.1) -> (-28.496, -73.3541)
  line L276 (-12.5, -84.1) -> (-6.5, -84.1)
  line L277 (-6.5, -84.1) -> (-6.5, -83.1)
  line L278 (-6.5, -83.1) -> (-12.5, -77.1)
  line L279 (-12.5, -77.1) -> (-12.5, -72.4023)
  arc A134 (-19.8023, -65.1) -> (-12.5, -72.4023) centre (-12.5, -65.1) ccw
  line L280 (-19.8023, -65.1) -> (-24.5, -65.1)
  line L281 (-24.5, -65.1) -> (-27.5, -62.1)
  line L282 (-27.5, -62.1) -> (-27.5, -52.1)
  line L283 (-27.5, -52.1) -> (-28.5, -52.1)
  line L284 (-28.5, -52.1) -> (-28.5, -61.1)
  line L285 (-28.5, -61.1) -> (-30.5, -59.1)
  line L286 (-30.5, -59.1) -> (-31.5, -59.1)
  line L287 (-31.5, -59.1) -> (-31.5, -65.1)
  arc A135 (-31.5, -65.1) -> (-12.5, -84.1) centre (-12.5, -65.1) ccw
  line L288 (62.7, 28.9) -> (31.2, 28.9)
  line L289 (31.2, 28.9) -> (62.7, 28.9)
  arc A136 (65.7, 25.9) -> (62.7, 28.9) centre (62.7, 25.9) ccw
  arc A137 (65.7, 25.9) -> (62.7, 28.9) centre (62.7, 25.9) ccw
  line L290 (93.9, -75.1) -> (0, -75.1)
  line L291 (0, -75.1) -> (93.9, -75.1)
  line L292 (-23.188, -59.3239) -> (-23.188, -62.3239)
  arc A138 (-23.188, -62.3239) -> (-20.188, -62.3239) centre (-21.688, -62.3239) ccw
  line L293 (-20.188, -62.3239) -> (-20.188, -59.3239)
  arc A139 (-20.188, -59.3239) -> (-23.188, -59.3239) centre (-21.688, -59.3239) ccw
  arc A140 (-27.4749, 32.8) -> (-31.5, 25.3) centre (-22.5, 25.3) ccw
  line L294 (-27.4749, 32.8) -> (-15.9888, 32.8)
  line L295 (-15.9888, 32.8) -> (-17.8764, 30.7591)
  arc A141 (-17.8764, 30.7591) -> (-15.9888, 31.4975) centre (-16.1, 29) ccw
  line L296 (-15.9888, 31.4975) -> (-15.9888, 32.8)
  line L297 (-15.9888, 32.8) -> (121.3749, 32.8)
  arc A142 (125.4, 25.3) -> (121.3749, 32.8) centre (116.4, 25.3) ccw
  line L298 (125.4, 25.3) -> (125.4, -65.1)
  arc A143 (106.4, -84.1) -> (125.4, -65.1) centre (106.4, -65.1) ccw
  line L299 (106.4, -84.1) -> (-12.5, -84.1)
  arc A144 (-31.5, -65.1) -> (-12.5, -84.1) centre (-12.5, -65.1) ccw
  line L300 (-31.5, -65.1) -> (-31.5, -25.2)
  line L301 (-31.5, -25.2) -> (-31.5, 25.3)
  line L302 (0, 4.1) -> (0, -75.1)
  line L303 (0, -75.1) -> (93.9, -75.1)
  line L304 (93.9, -75.1) -> (93.9, 4.1)
  line L305 (93.9, 4.1) -> (0, 4.1)
  circle A145 centre (102.6547, -56.4453) radius 2.35
  circle A146 centre (117.6453, -56.4453) radius 2.35
  circle A147 centre (110.15, -33.95) radius 3.85
  circle A148 centre (102.65, -41.45) radius 3.85
  circle A149 centre (117.65, -41.45) radius 3.85
  circle A150 centre (110.15, -48.95) radius 3.85
  arc A151 (47.45, -79.6) -> (46.45, -79.6) centre (46.95, -79.6) ccw
  line L306 (46.45, -79.6) -> (45.65, -79.6)
  arc A152 (45.65, -79.6) -> (45.65, -80.6) centre (45.65, -80.1) ccw
  line L307 (45.65, -80.6) -> (46.45, -80.6)
  arc A153 (46.45, -80.6) -> (47.45, -80.6) centre (46.95, -80.6) ccw
  line L308 (47.45, -80.6) -> (48.25, -80.6)
  arc A154 (48.25, -80.6) -> (48.25, -79.6) centre (48.25, -80.1) ccw
  line L309 (48.25, -79.6) -> (47.45, -79.6)
  line L310 (98.8996, 12.7) -> (88.8996, 12.7)
  arc A155 (88.8996, 12.7) -> (88.9, 10.7) centre (88.9, 11.7) ccw
  line L311 (88.9, 10.7) -> (98.9, 10.7)
  arc A156 (98.9, 10.7) -> (98.8996, 12.7) centre (98.9, 11.7) ccw
  line L312 (85.7348, 14.7) -> (102.0652, 14.7)
  arc A157 (102.0652, 14.7) -> (102.0652, 16.7) centre (102.0652, 15.7) ccw
  line L313 (102.0652, 16.7) -> (85.7348, 16.7)
  arc A158 (85.7348, 16.7) -> (85.7348, 14.7) centre (85.7348, 15.7) ccw
  arc A159 (102.0652, 22.7) -> (102.0652, 24.7) centre (102.0652, 23.7) ccw
  line L314 (102.0652, 24.7) -> (85.7348, 24.7)
  arc A160 (85.7348, 24.7) -> (85.7348, 22.7) centre (85.7348, 23.7) ccw
  line L315 (85.7348, 22.7) -> (102.0652, 22.7)
  arc A161 (98.9004, 26.7) -> (98.9, 28.7) centre (98.9, 27.7) ccw
  line L316 (98.9, 28.7) -> (88.9, 28.7)
  arc A162 (88.9, 28.7) -> (88.8996, 26.7) centre (88.9, 27.7) ccw
  line L317 (88.8996, 26.7) -> (98.9004, 26.7)
  arc A163 (102.9, 18.7) -> (102.9, 20.7) centre (102.9, 19.7) ccw
  line L318 (102.9, 20.7) -> (84.9, 20.7)
  arc A164 (84.9, 20.7) -> (84.9, 18.7) centre (84.9, 19.7) ccw
  line L319 (84.9, 18.7) -> (102.9, 18.7)
  line L320 (-8.1652, 14.7) -> (8.1652, 14.7)
  arc A165 (8.1652, 14.7) -> (8.1652, 16.7) centre (8.1652, 15.7) ccw
  line L321 (8.1652, 16.7) -> (-8.1652, 16.7)
  arc A166 (-8.1652, 16.7) -> (-8.1652, 14.7) centre (-8.1652, 15.7) ccw
  arc A167 (-9, 20.7) -> (-9, 18.7) centre (-9, 19.7) ccw
  line L322 (-9, 18.7) -> (9, 18.7)
  arc A168 (9, 18.7) -> (9, 20.7) centre (9, 19.7) ccw
  line L323 (9, 20.7) -> (-9, 20.7)
  line L324 (8.1652, 24.7) -> (-8.1652, 24.7)
  arc A169 (-8.1652, 24.7) -> (-8.1652, 22.7) centre (-8.1652, 23.7) ccw
  line L325 (-8.1652, 22.7) -> (8.1652, 22.7)
  arc A170 (8.1652, 22.7) -> (8.1652, 24.7) centre (8.1652, 23.7) ccw
  arc A171 (-5, 28.7) -> (-5.0004, 26.7) centre (-5, 27.7) ccw
  line L326 (-5.0004, 26.7) -> (4.9996, 26.7)
  arc A172 (4.9996, 26.7) -> (5, 28.7) centre (5, 27.7) ccw
  line L327 (5, 28.7) -> (-5, 28.7)
  arc A173 (-5.0004, 12.7) -> (-5, 10.7) centre (-5, 11.7) ccw
  line L328 (-5, 10.7) -> (5, 10.7)
  arc A174 (5, 10.7) -> (5.0004, 12.7) centre (5, 11.7) ccw
  line L329 (5.0004, 12.7) -> (-5.0004, 12.7)
  line L330 (34.2, 32.4) -> (34.2, 30.4)
  line L331 (34.2, 30.4) -> (27.2, 30.4)
  line L332 (27.2, 30.4) -> (27.2, 10)
  arc A175 (27.2, 10) -> (29.2, 8) centre (29.2, 10) ccw
  line L333 (29.2, 8) -> (64.7, 8)
  arc A176 (64.7, 8) -> (66.7, 10) centre (64.7, 10) ccw
  line L334 (66.7, 10) -> (66.7, 30.4)
  line L335 (66.7, 30.4) -> (59.7, 30.4)
  line L336 (59.7, 30.4) -> (59.7, 32.4)
  line L337 (59.7, 32.4) -> (34.2, 32.4)
  line L338 (-13, -32.2) -> (-19.5, -32.2)
  line L339 (-19.5, -32.2) -> (-19.5, -38.2)
  line L340 (-19.5, -38.2) -> (-25.5, -38.2)
  line L341 (-25.5, -38.2) -> (-25.5, -44.7)
  line L342 (-25.5, -44.7) -> (-19.5, -44.7)
  line L343 (-19.5, -44.7) -> (-19.5, -50.7)
  line L344 (-19.5, -50.7) -> (-13, -50.7)
  line L345 (-13, -50.7) -> (-13, -44.7)
  line L346 (-13, -44.7) -> (-7, -44.7)
  line L347 (-7, -44.7) -> (-7, -38.2)
  line L348 (-7, -38.2) -> (-13, -38.2)
  line L349 (-13, -38.2) -> (-13, -32.2)
  circle A177 centre (-10.8119, -62.3239) radius 1.5
  line L350 (65.7, 12.5) -> (65.7, 25.9)
  line L351 (65.7, 25.9) -> (65.7, 12.5)
  circle A178 centre (84.4, -5) radius 2.5
  circle A179 centre (84.4, -5) radius 2.5
  arc A180 (28.2, 12.5) -> (31.2, 9.5) centre (31.2, 12.5) ccw
  arc A181 (28.2, 12.5) -> (31.2, 9.5) centre (31.2, 12.5) ccw
  line L352 (-7, -3.65) -> (-2, -3.65)
  line L353 (-2, -3.65) -> (-7, -3.65)
  line L354 (27.2, 4.1) -> (0, 4.1)
  line L355 (0, 4.1) -> (93.9, 4.1)
  line L356 (93.9, 4.1) -> (66.7, 4.1)
  line L357 (66.7, 4.1) -> (27.2, 4.1)
  circle A182 centre (80.15, -44.4) radius 2.5
  circle A183 centre (80.15, -44.4) radius 2.5
  line L358 (27.2, 33.9) -> (27.2, 4.5)
  line L359 (27.2, 4.5) -> (66.7, 4.5)
  line L360 (66.7, 4.5) -> (66.7, 33.9)
  line L361 (66.7, 33.9) -> (27.2, 33.9)
  arc A184 (31.2, 28.9) -> (28.2, 25.9) centre (31.2, 25.9) ccw
  arc A185 (31.2, 28.9) -> (28.2, 25.9) centre (31.2, 25.9) ccw
  line L362 (24.5, -83.65) -> (24.5, -81.15)
  line L363 (24.5, -81.15) -> (24.5, -83.65)
  line L364 (83.1181, 15.7) -> (80.4836, 15.7)
  arc A186 (80.4836, 15.7) -> (80.4836, 23.7) centre (93.9, 19.7) ccw
  line L365 (80.4836, 23.7) -> (83.1181, 23.7)
  arc A187 (83.1181, 15.7) -> (83.1181, 23.7) centre (93.9, 19.7) ccw
  line L366 (-24.0635, 35.177) -> (-22.5, 35.177)
  line L367 (-22.5, 35.177) -> (-22.5, 35.3)
  line L368 (-22.5, 35.3) -> (116.4, 35.3)
  line L369 (116.4, 35.3) -> (116.4, 35.177)
  line L370 (116.4, 35.177) -> (117.9635, 35.177)
  spline S4 degree 3 poles (120.0657, 34.6039) (119.5111, 34.8224) (118.9454, 34.9877) (118.2417, 35.13) (118.1027, 35.155) (117.9635, 35.177) knots -0.429091 -0.429091 -0.429091 -0.429091 -0.227456 -0.227456 -0.177677 -0.177677 -0.177677 -0.177677
  spline S5 degree 3 poles (121.3749, 32.8) (121.4016, 32.8) (121.4257, 32.8021) (121.4681, 32.811) (121.489, 32.8182) (121.521, 32.8394) (121.5326, 32.8506) (121.5513, 32.8783) (121.5579, 32.8938) (121.5687, 32.9351) (121.5705, 32.9623) (121.568, 33.0372) (121.5571, 33.0944) (121.5047, 33.2719) (121.442, 33.4168) (121.2247, 33.772) (121.0595, 33.976) (120.605, 34.3502) (120.3486, 34.4924) (120.0657, 34.6039) knots 1.719139 1.719139 1.719139 1.719139 1.741292 1.741292 1.762806 1.762806 1.778603 1.778603 1.794207 1.794207 1.817491 1.817491 1.860621 1.860621 1.939646 1.939646 2.038469 2.038469 2.13754 2.13754 2.13754 2.13754
  line L371 (121.3749, 32.8) -> (-15.9888, 32.8)
  line L372 (-15.9888, 32.8) -> (-27.4749, 32.8)
  spline S6 degree 3 poles (-26.1657, 34.6039) (-26.5128, 34.4672) (-26.796, 34.2925) (-27.2865, 33.8432) (-27.4579, 33.5817) (-27.6034, 33.268) (-27.6354, 33.1786) (-27.6643, 33.054) (-27.6732, 32.9982) (-27.6666, 32.9257) (-27.6619, 32.9031) (-27.6451, 32.8674) (-27.6355, 32.8538) (-27.6103, 32.831) (-27.5957, 32.8224) (-27.558, 32.8077) (-27.5332, 32.803) (-27.496, 32.8003) (-27.4857, 32.8) (-27.4749, 32.8) knots 0.503021 0.503021 0.503021 0.503021 0.608582 0.608582 0.725176 0.725176 0.775103 0.775103 0.805659 0.805659 0.818798 0.818798 0.828249 0.828249 0.837394 0.837394 0.849434 0.849434 0.853721 0.853721 0.853721 0.853721
  spline S7 degree 3 poles (-24.0635, 35.177) (-24.2027, 35.155) (-24.3417, 35.13) (-25.0454, 34.9877) (-25.6111, 34.8224) (-26.1657, 34.6039) knots 0.177677 0.177677 0.177677 0.177677 0.227456 0.227456 0.429091 0.429091 0.429091 0.429091
  line L373 (18, -81.15) -> (18, -77.2)
  line L374 (18, -77.2) -> (10.5, -77.2)
  line L375 (10.5, -77.2) -> (10.5, -81.15)
  arc A188 (5.5, -81.15) -> (10.5, -81.15) centre (8, -81.15) ccw
  line L376 (5.5, -81.15) -> (5.5, -77.2)
  line L377 (5.5, -77.2) -> (-2, -77.2)
  line L378 (-2, -77.2) -> (-2, -85.1)
  line L379 (-2, -85.1) -> (75.9, -85.1)
  line L380 (75.9, -85.1) -> (75.9, -81.15)
  arc A189 (70.9, -81.15) -> (75.9, -81.15) centre (73.4, -81.15) ccw
  line L381 (70.9, -81.15) -> (70.9, -77.2)